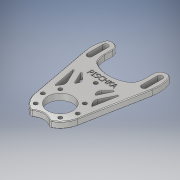
# Autodesk Inventor part: Motor Holder v3
Saved by Autodesk Inventor 2019.4 (Build 234330000, 330)
## iProperties
Created: 2019-03-01
Part Number: Motor Holder v3
Material: Aluminum 6061-AHC
Document SubType Name: Modeling
Designer: Petar
Density: 2.7 g/cm^3
Appearance: Aluminum - Dark
Mass: 26.5004 g
Surface Area: 70.5339 cm^2
Volume: 9.81495 cm^3
Author: Petar
Autodesk Inventor part; units mm, degrees
ref_plane "YZ Plane" through (0, 0, 0) normal (1, 0, 0) x (0, 1, 0)
ref_plane "XZ Plane" through (0, 0, 0) normal (0, 1, 0) x (-1, 0, 0)
ref_plane "XY Plane" through (0, 0, 0) normal (0, 0, 1) x (1, 0, 0)
sketch "Sketch1" plane through (0, 0, 0) normal (0, 1, 0) x (-1, 0, 0)
  line L0 (0, 0) -> (0, 51) construction
  circle A0 centre (0, 51) radius 10
  line L1 (16, -6.25) -> (16, 0)
  line L2 (21.5, 19.954117) -> (21.5, -14.045883) construction
  line L3 (-21.5, 18) -> (-21.5, -16) construction
  circle A1 centre (21.5, 3.5) radius 1.75 construction
  circle A2 centre (21.5, -3.5) radius 1.75 construction
  circle A3 centre (-21.5, 3.5) radius 1.75 construction
  circle A4 centre (-21.5, -3.5) radius 1.75 construction
  line L4 (-16, -6.25) -> (-16, 0)
  line L5 (21.5, 6.25) -> (21.5, -6.25) construction
  line L6 (19.45, 6.25) -> (19.45, -6.25)
  line L7 (23.55, -6.25) -> (23.55, 6.25)
  arc A5 (23.55, 6.25) -> (19.45, 6.25) centre (21.5, 6.25) ccw
  arc A6 (19.45, -6.25) -> (23.55, -6.25) centre (21.5, -6.25) ccw
  line L8 (-19.45, 6.25) -> (-19.45, -6.25)
  line L9 (-23.55, -6.25) -> (-23.55, 6.25)
  arc A7 (-19.45, 6.25) -> (-23.55, 6.25) centre (-21.5, 6.25) ccw
  arc A8 (-23.55, -6.25) -> (-19.45, -6.25) centre (-21.5, -6.25) ccw
  arc A9 (14.562609, 41.295341) -> (17.19371, 54.259804) centre (0, 51) ccw construction
  arc A10 (16, -6.25) -> (24.816002, -10.637953) centre (21.5, -6.25) ccw
  arc A11 (-24.816002, -10.637953) -> (-16, -6.25) centre (-21.5, -6.25) ccw
  line L10 (17.19371, 54.259804) -> (26.527439, 5.029412)
  line L11 (-17.19371, 54.259804) -> (-26.527439, 5.029412)
  circle A12 centre (0, 51) radius 13.75 construction
  circle A13 centre (9.722718, 60.722718) radius 1.5
  circle A14 centre (9.722718, 41.277282) radius 1.5
  line L12 (0, 51) -> (9.722718, 60.722718) construction
  line L13 (9.722718, 41.277282) -> (0, 51) construction
  circle A15 centre (-9.722718, 60.722718) radius 1.5
  circle A16 centre (-9.722718, 41.277282) radius 1.5
  circle A17 centre (13.75, 51) radius 1.5
  line L14 (13.75, 51) -> (0, 51) construction
  circle A18 centre (-13.75, 51) radius 1.5
  circle A19 centre (0, 22.976561) radius 1.5
  line L15 (14.562609, 41.295341) -> (18.699293, 19.476561)
  arc A20 (17.19371, 54.259804) -> (-17.19371, 54.259804) centre (0, 51) ccw
  arc A21 (-17.19371, 54.259804) -> (-14.562609, 41.295341) centre (0, 51) ccw construction
  line L16 (-14.562609, 41.295341) -> (-18.699293, 19.476561)
  line L17 (7.5, 66.811388) -> (0, 61) construction
  line L18 (0, 61) -> (-7.5, 66.811388) construction
  spline S0 degree 2 poles (7.5, 66.811388) (0, 61) (-7.5, 66.811388) knots 1 1 1 2 2 2
  line L19 (7.5, 66.811388) -> (-7.5, 66.811388) construction
  line L20 (18.699293, 19.476561) -> (-18.699293, 19.476561) construction
  line L21 (18.699293, 19.476561) -> (11.899653, 33.58283)
  line L22 (14.562609, 41.295341) -> (12.187745, 37.73167)
  arc A22 (12.187745, 37.73167) -> (11.899653, 33.58283) centre (15.679416, 35.404788) ccw
  line L23 (-18.699293, 19.476561) -> (-11.899653, 33.58283)
  line L24 (-14.562609, 41.295341) -> (-12.187745, 37.73167)
  arc A23 (-11.899653, 33.58283) -> (-12.187745, 37.73167) centre (-15.679416, 35.404788) ccw
  line L25 (14.258838, 19.476561) -> (8.283423, 31.872924)
  line L26 (14.258838, 19.476561) -> (7.634459, 25.898167)
  line L27 (8.283423, 31.872924) -> (7.173527, 30.207438)
  arc A24 (7.173527, 30.207438) -> (7.634459, 25.898167) centre (9.991429, 28.329562) ccw
  line L28 (-14.258838, 19.476561) -> (-8.283423, 31.872924)
  line L29 (-14.258838, 19.476561) -> (-7.634459, 25.898167)
  line L30 (-8.283423, 31.872924) -> (-7.173527, 30.207438)
  arc A25 (-7.634459, 25.898167) -> (-7.173527, 30.207438) centre (-9.991429, 28.329562) ccw
  arc A26 (24.816002, -10.637953) -> (27, 0) centre (0, 0) ccw
  arc A27 (-24.816002, -10.637953) -> (24.816002, -10.637953) centre (0, 0) ccw construction
  arc A28 (-10.301604, 24.957503) -> (-26.527439, 5.029412) centre (0, 0) ccw construction
  line L31 (21.5, -11.75) -> (-21.5, -11.75) construction
  line L32 (-21.213203, 68.5) -> (25, 68.5) construction
  line L33 (0, 61) -> (0, 61) construction
  arc A29 (13.760985, 8.163043) -> (-13.760985, 8.163043) centre (0, -11.5) ccw
  line L34 (13.760985, 8.163043) -> (-13.760985, 8.163043) construction
  arc A30 (16, 0) -> (13.760985, 8.163043) centre (0, 0) ccw
  arc A31 (-13.760985, 8.163043) -> (-16, 0) centre (0, 0) ccw
  arc A32 (27, 0) -> (26.527439, 5.029412) centre (0, 0) ccw
  arc A33 (-27, 0) -> (-24.816002, -10.637953) centre (0, 0) ccw
  arc A34 (-26.527439, 5.029412) -> (-27, 0) centre (0, 0) ccw
  arc A35 (26.527439, 5.029412) -> (-11.984726, 24.194345) centre (0, 0) ccw construction
  line L35 (16, 0) -> (-16, 0) construction
  point P0 (21.5, 0)
  point P1 (0, 12.5)
  dimension "d1" = 20
  dimension "d0" = 51
  dimension "d3" = 3.5
  dimension "d4" = 3.5
  dimension "d5" = 7
  dimension "d9" = 3.5
  dimension "d11" = 32
  dimension "d15" = 4.1
  dimension "d24" = 3
  dimension "d25" = 3
  dimension "d27" = 45
  dimension "d29" = 3
  dimension "d30" = 3
  dimension "d50" = 15
  dimension "d53" = 27
  dimension "d75" = 80.25
  dimension "d76" = 7.5
  dimension "d77" = 3.75
  dimension "d78" = 0
  dimension "d81" = 6.25
  dimension "d82" = 12.5
  dimension "d85" = 5
  dimension "d86" = 4
  dimension "d98" = 15
  dimension "d99" = 24
  dimension "d101" = 43
  dimension "d104" = 2
  constraints: 70 end point, 58 point on circle, 35 centre point, 26 symmetric about line, 19 tangent, 13 point on line, 7 coincident, 5 horizontal, 5 vertical, 3 parallel, 2 perpendicular, 1 collinear, 1 midpoint, 1 vertical alignment, 16 other
  measures "d0" distance of L0.start L0.end
  measures "d3" diameter of A1
  measures "d4" diameter of A2
  measures "d5" distance of A2.centre A1.centre
  measures "d9" vertical distance of L0.start A1.centre
  measures "d11" distance between parallel lines of L4 L1
  measures "d15" distance between parallel lines of L6 L7
  measures "d24" diameter of A13
  measures "d25" diameter of A14
  measures "d27" angle of L0 L13
  measures "d29" diameter of A17
  measures "d30" diameter of A19
  measures "d50" distance of L17.start L18.end
  measures "d53" radius of A26
  measures "d75" distance between parallel lines of L31 L32
  measures "d78" distance of L33.start L33.end
  measures "d81" vertical distance of L5.start point (0, 12.5)
  measures "d82" distance of L5.end L5.start
  measures "d85" distance between parallel lines of L10 L15
  measures "d86" distance between parallel lines of L21 L25
  measures "d98" angle of L15 L21
  measures "d99" radius of A29
  measures "d101" distance of A4.centre A2.centre
  measures "d104" distance edge to line of A19 L20
extrude "Extrusion3" add sketch "Sketch1" along normal blind 5 contours L1 A30 A29 A31 L4 A11 A33 A34 L11 A20 S0 L10 A32 A26 A10
thread "Thread1" size "M3x0.5" class "6H" standard "ANSI Metric M Profile" full length
thread "Thread2" size "M3x0.5" class "6H" standard "ANSI Metric M Profile" full length
thread "Thread3" size "M3x0.5" class "6H" standard "ANSI Metric M Profile" full length
thread "Thread4" size "M3x0.5" class "6H" standard "ANSI Metric M Profile" full length
thread "Thread5" size "M3x0.5" class "6H" standard "ANSI Metric M Profile" full length
thread "Thread6" size "M3x0.5" class "6H" standard "ANSI Metric M Profile" full length
thread "Thread7" size "M3x0.5" class "6H" standard "ANSI Metric M Profile" full length
sketch "Sketch3" plane through (0, 5, 0) normal (0, 1, 0) x (1, 0, 0)
  line L0 (-12.5, -14.976561) -> (12.5, -14.976561) construction
  line L1 (12.5, -14.976561) -> (12.5, -19.976561) construction
  line L2 (12.5, -19.976561) -> (-12.5, -19.976561) construction
  line L3 (-12.5, -19.976561) -> (-12.5, -14.976561) construction
  line L4 (0, 0) -> (0, -51) construction
  circle A0 centre (0, -22.976561) radius 1.5
  circle A1 centre (0, -51) radius 10 construction
  arc A2 (-24.816002, 10.637953) -> (-26.527439, -5.029412) centre (0, 0) ccw construction
  spline S0 degree 2 poles (-7.943274, -16.682396) (-7.943274, -16.941715) (-8.128039, -17.40849) (-8.293355, -17.570565) knots 0 0 0 1 2 2 2
  spline S1 degree 2 poles (-8.293355, -17.570565) (-8.500811, -17.774779) (-9.061589, -17.985475) (-9.489465, -17.985475) knots 0 0 0 1 2 2 2
  line L5 (-9.489465, -17.985475) -> (-9.940033, -17.985475)
  line L6 (-9.940033, -17.985475) -> (-9.940033, -19.476561)
  line L7 (-9.940033, -19.476561) -> (-10.471637, -19.476561)
  line L8 (-10.471637, -19.476561) -> (-10.471637, -15.476561)
  line L9 (-10.471637, -15.476561) -> (-9.466775, -15.476561)
  spline S2 degree 2 poles (-9.466775, -15.476561) (-9.110211, -15.476561) (-8.611021, -15.593255) (-8.419773, -15.726156) knots 0 0 0 1 2 2 2
  spline S3 degree 2 poles (-8.419773, -15.726156) (-8.19611, -15.878506) (-7.943274, -16.348522) (-7.943274, -16.682396) knots 0 0 0 1 2 2 2
  spline S4 degree 2 poles (-8.497569, -16.698603) (-8.497569, -16.491148) (-8.640195, -16.186448) (-8.786062, -16.089203) knots 0 0 0 1 2 2 2
  spline S5 degree 2 poles (-8.786062, -16.089203) (-8.91248, -16.004924) (-9.249595, -15.936853) (-9.49919, -15.936853) knots 0 0 0 1 2 2 2
  line L10 (-9.49919, -15.936853) -> (-9.940033, -15.936853)
  line L11 (-9.940033, -15.936853) -> (-9.940033, -17.531667)
  line L12 (-9.940033, -17.531667) -> (-9.576986, -17.531667)
  spline S6 degree 2 poles (-9.576986, -17.531667) (-9.252837, -17.531667) (-8.854133, -17.427939) (-8.724474, -17.291796) knots 0 0 0 1 2 2 2
  spline S7 degree 2 poles (-8.724474, -17.291796) (-8.604538, -17.171861) (-8.497569, -16.889851) (-8.497569, -16.698603) knots 0 0 0 1 2 2 2
  line L13 (-6.04376, -19.476561) -> (-7.593193, -19.476561)
  line L14 (-7.593193, -19.476561) -> (-7.593193, -19.068133)
  line L15 (-7.593193, -19.068133) -> (-7.084279, -19.068133)
  line L16 (-7.084279, -19.068133) -> (-7.084279, -15.884989)
  line L17 (-7.084279, -15.884989) -> (-7.593193, -15.884989)
  line L18 (-7.593193, -15.884989) -> (-7.593193, -15.476561)
  line L19 (-7.593193, -15.476561) -> (-6.04376, -15.476561)
  line L20 (-6.04376, -15.476561) -> (-6.04376, -15.884989)
  line L21 (-6.04376, -15.884989) -> (-6.552674, -15.884989)
  line L22 (-6.552674, -15.884989) -> (-6.552674, -19.068133)
  line L23 (-6.552674, -19.068133) -> (-6.04376, -19.068133)
  line L24 (-6.04376, -19.068133) -> (-6.04376, -19.476561)
  spline S8 degree 2 poles (-4.270665, -19.547874) (-4.705025, -19.547874) (-5.314425, -19.366351) (-5.583469, -19.236691) knots 0 0 0 1 2 2 2
  line L25 (-5.583469, -19.236691) -> (-5.583469, -18.568944)
  line L26 (-5.583469, -18.568944) -> (-5.544571, -18.568944)
  spline S9 degree 2 poles (-5.544571, -18.568944) (-5.28201, -18.815297) (-4.617504, -19.087582) (-4.309563, -19.087582) knots 0 0 0 1 2 2 2
  spline S10 degree 2 poles (-4.309563, -19.087582) (-3.86872, -19.087582) (-3.418153, -18.721294) (-3.418153, -18.419835) knots 0 0 0 1 2 2 2
  spline S11 degree 2 poles (-3.418153, -18.419835) (-3.418153, -18.179965) (-3.654781, -17.881748) (-3.910859, -17.807193) knots 0 0 0 1 2 2 2
  spline S12 degree 2 poles (-3.910859, -17.807193) (-4.095624, -17.75533) (-4.403566, -17.684017) (-4.633712, -17.62567) knots 0 0 0 1 2 2 2
  spline S13 degree 2 poles (-4.633712, -17.62567) (-4.841167, -17.570565) (-5.168558, -17.405249) (-5.294976, -17.272347) knots 0 0 0 1 2 2 2
  spline S14 degree 2 poles (-5.294976, -17.272347) (-5.418153, -17.139446) (-5.554295, -16.782882) (-5.554295, -16.549495) knots 0 0 0 1 2 2 2
  spline S15 degree 2 poles (-5.554295, -16.549495) (-5.554295, -16.063271) (-4.795786, -15.405248) (-4.209076, -15.405248) knots 0 0 0 1 2 2 2
  spline S16 degree 2 poles (-4.209076, -15.405248) (-3.871961, -15.405248) (-3.275527, -15.53815) (-3.019449, -15.664568) knots 0 0 0 1 2 2 2
  line L27 (-3.019449, -15.664568) -> (-3.019449, -16.2999)
  line L28 (-3.019449, -16.2999) -> (-3.058347, -16.2999)
  spline S17 degree 2 poles (-3.058347, -16.2999) (-3.249595, -16.12486) (-3.846029, -15.86554) (-4.17342, -15.86554) knots 0 0 0 1 2 2 2
  spline S18 degree 2 poles (-4.17342, -15.86554) (-4.54295, -15.86554) (-5, -16.21238) (-5, -16.49439) knots 0 0 0 1 2 2 2
  spline S19 degree 2 poles (-5, -16.49439) (-5, -16.747226) (-4.730956, -17.048684) (-4.47812, -17.116756) knots 0 0 0 1 2 2 2
  spline S20 degree 2 poles (-4.47812, -17.116756) (-4.309563, -17.162137) (-3.820097, -17.27883) (-3.658023, -17.327453) knots 0 0 0 1 2 2 2
  spline S21 degree 2 poles (-3.658023, -17.327453) (-3.246354, -17.453871) (-2.863858, -17.962785) (-2.863858, -18.335556) knots 0 0 0 1 2 2 2
  spline S22 degree 2 poles (-2.863858, -18.335556) (-2.863858, -18.572185) (-3.055106, -19.025994) (-3.226905, -19.184827) knots 0 0 0 1 2 2 2
  spline S23 degree 2 poles (-3.226905, -19.184827) (-3.418153, -19.359868) (-3.904376, -19.547874) (-4.270665, -19.547874) knots 0 0 0 1 2 2 2
  spline S24 degree 2 poles (-0.76013, -19.547874) (-1.149109, -19.547874) (-1.807131, -19.285313) (-2.047002, -19.022753) knots 0 0 0 1 2 2 2
  spline S25 degree 2 poles (-2.047002, -19.022753) (-2.286872, -18.763433) (-2.549433, -17.985475) (-2.549433, -17.479803) knots 0 0 0 1 2 2 2
  spline S26 degree 2 poles (-2.549433, -17.479803) (-2.549433, -16.977372) (-2.293355, -16.231829) (-2.050243, -15.956302) knots 0 0 0 1 2 2 2
  spline S27 degree 2 poles (-2.050243, -15.956302) (-1.810373, -15.687258) (-1.155592, -15.405248) (-0.750405, -15.405248) knots 0 0 0 1 2 2 2
  spline S28 degree 2 poles (-0.750405, -15.405248) (-0.549433, -15.405248) (-0.19611, -15.463595) (-0.047002, -15.508976) knots 0 0 0 1 2 2 2
  spline S29 degree 2 poles (-0.047002, -15.508976) (0.082658, -15.551116) (0.351702, -15.671051) (0.484603, -15.742364) knots 0 0 0 1 2 2 2
  line L29 (0.484603, -15.742364) -> (0.484603, -16.384179)
  line L30 (0.484603, -16.384179) -> (0.442463, -16.384179)
  spline S30 degree 2 poles (0.442463, -16.384179) (0.371151, -16.319349) (0.150729, -16.137825) (-0.008104, -16.050305) knots 0 0 0 1 2 2 2
  spline S31 degree 2 poles (-0.008104, -16.050305) (-0.160454, -15.966026) (-0.520259, -15.859057) (-0.753647, -15.859057) knots 0 0 0 1 2 2 2
  spline S32 degree 2 poles (-0.753647, -15.859057) (-1.009725, -15.859057) (-1.466775, -16.069754) (-1.638574, -16.270727) knots 0 0 0 1 2 2 2
  spline S33 degree 2 poles (-1.638574, -16.270727) (-1.807131, -16.474941) (-1.995138, -17.094065) (-1.995138, -17.479803) knots 0 0 0 1 2 2 2
  spline S34 degree 2 poles (-1.995138, -17.479803) (-1.995138, -17.891472) (-1.797407, -18.484665) (-1.625608, -18.688879) knots 0 0 0 1 2 2 2
  spline S35 degree 2 poles (-1.625608, -18.688879) (-1.45705, -18.88661) (-1.006483, -19.087582) (-0.753647, -19.087582) knots 0 0 0 1 2 2 2
  spline S36 degree 2 poles (-0.753647, -19.087582) (-0.523501, -19.087582) (-0.131281, -18.97413) (0.02107, -18.889851) knots 0 0 0 1 2 2 2
  spline S37 degree 2 poles (0.02107, -18.889851) (0.166937, -18.805573) (0.384117, -18.630532) (0.445705, -18.568944) knots 0 0 0 1 2 2 2
  line L31 (0.445705, -18.568944) -> (0.484603, -18.568944)
  line L32 (0.484603, -18.568944) -> (0.484603, -19.204276)
  spline S38 degree 2 poles (0.484603, -19.204276) (0.351702, -19.265864) (0.118314, -19.379317) (-0.047002, -19.43118) knots 0 0 0 1 2 2 2
  spline S39 degree 2 poles (-0.047002, -19.43118) (-0.222042, -19.489527) (-0.520259, -19.547874) (-0.76013, -19.547874) knots 0 0 0 1 2 2 2
  line L33 (3.884927, -19.476561) -> (3.353322, -19.476561)
  line L34 (3.353322, -19.476561) -> (3.353322, -17.518701)
  line L35 (3.353322, -17.518701) -> (1.512155, -17.518701)
  line L36 (1.512155, -17.518701) -> (1.512155, -19.476561)
  line L37 (1.512155, -19.476561) -> (0.980551, -19.476561)
  line L38 (0.980551, -19.476561) -> (0.980551, -15.476561)
  line L39 (0.980551, -15.476561) -> (1.512155, -15.476561)
  line L40 (1.512155, -15.476561) -> (1.512155, -17.045443)
  line L41 (1.512155, -17.045443) -> (3.353322, -17.045443)
  line L42 (3.353322, -17.045443) -> (3.353322, -15.476561)
  line L43 (3.353322, -15.476561) -> (3.884927, -15.476561)
  line L44 (3.884927, -15.476561) -> (3.884927, -19.476561)
  line L45 (7.612642, -19.476561) -> (6.922204, -19.476561)
  line L46 (6.922204, -19.476561) -> (5.460292, -17.615945)
  line L47 (5.460292, -17.615945) -> (5.226904, -17.878506)
  line L48 (5.226904, -17.878506) -> (5.226904, -19.476561)
  line L49 (5.226904, -19.476561) -> (4.6953, -19.476561)
  line L50 (4.6953, -19.476561) -> (4.6953, -15.476561)
  line L51 (4.6953, -15.476561) -> (5.226904, -15.476561)
  line L52 (5.226904, -15.476561) -> (5.226904, -17.314487)
  line L53 (5.226904, -17.314487) -> (6.867099, -15.476561)
  line L54 (6.867099, -15.476561) -> (7.515397, -15.476561)
  line L55 (7.515397, -15.476561) -> (5.858995, -17.262623)
  line L56 (5.858995, -17.262623) -> (7.612642, -19.476561)
  line L57 (7.49919, -19.476561) -> (8.84765, -15.476561)
  line L58 (8.84765, -15.476561) -> (9.502431, -15.476561)
  line L59 (9.502431, -15.476561) -> (10.850891, -19.476561)
  line L60 (10.850891, -19.476561) -> (10.290113, -19.476561)
  line L61 (10.290113, -19.476561) -> (9.927066, -18.358247)
  line L62 (9.927066, -18.358247) -> (8.400324, -18.358247)
  line L63 (8.400324, -18.358247) -> (8.037277, -19.476561)
  line L64 (8.037277, -19.476561) -> (7.49919, -19.476561)
  line L65 (9.781199, -17.904438) -> (9.162075, -16.021132)
  line L66 (9.162075, -16.021132) -> (8.546191, -17.904438)
  line L67 (8.546191, -17.904438) -> (9.781199, -17.904438)
  dimension "d68" = 3
  dimension "d69" = 5
  dimension "d70" = 25
  constraints: 2 coincident, 2 end point, 1 vertical, 3 other
  measures "d68" distance from line of L2 A0.centre
  measures "d69" distance between parallel lines of L0 L2
  measures "d70" distance between parallel lines of L3 L1
emboss "Emboss1" sketch "Sketch3" operation cut depth 0.2 direction (0, -1, 0) contours S0 S1 L5 L6 L7 L8 L9 S2 S3 | L13 L14 L15 L16 L17 L18 L19 L20 L21 L22 L23 L24 | S8 L25 L26 S9 S10 S11 S12 S13 S14 S15 S16 L27 L28 S17 S18 S19 S20 S21 S22 S23 | S24 S25 S26 S27 S28 S29 L29 L30 S30 S31 S32 S33 S34 S35 S36 S37 L31 L32 S38 S39 | L33 L34 L35 L36 L37 L38 L39 L40 L41 L42 L43 L44 | L45 L57 L56 | L56 L57 L58 L59 L60 L61 L62 L63 L64 | L45 L46 L47 L48 L49 L50 L51 L52 L53 L54 L55 L56 L57
sketch "Sketch4" plane through (0, 0, 0) normal (0, -1, 0) x (1, 0, 0)
  circle A0 centre (0, 22.976561) radius 1.5
  line L0 (12.5, 14.976561) -> (-12.5, 14.976561) construction
  line L1 (-12.5, 14.976561) -> (-12.5, 19.976561) construction
  line L2 (-12.5, 19.976561) -> (12.5, 19.976561) construction
  line L3 (12.5, 19.976561) -> (12.5, 14.976561) construction
  circle A1 centre (0, 51) radius 10 construction
  arc A2 (24.816002, -10.637953) -> (26.527439, 5.029412) centre (0, 0) ccw construction
  line L4 (0, 0) -> (0, 51) construction
  spline S0 degree 2 poles (7.943274, 16.682396) (7.943274, 16.941715) (8.128039, 17.40849) (8.293355, 17.570565) knots 0 0 0 1 2 2 2
  spline S1 degree 2 poles (8.293355, 17.570565) (8.500811, 17.774779) (9.061589, 17.985475) (9.489465, 17.985475) knots 0 0 0 1 2 2 2
  line L5 (9.489465, 17.985475) -> (9.940033, 17.985475)
  line L6 (9.940033, 17.985475) -> (9.940033, 19.476561)
  line L7 (9.940033, 19.476561) -> (10.471637, 19.476561)
  line L8 (10.471637, 19.476561) -> (10.471637, 15.476561)
  line L9 (10.471637, 15.476561) -> (9.466775, 15.476561)
  spline S2 degree 2 poles (9.466775, 15.476561) (9.110211, 15.476561) (8.611021, 15.593255) (8.419773, 15.726156) knots 0 0 0 1 2 2 2
  spline S3 degree 2 poles (8.419773, 15.726156) (8.19611, 15.878506) (7.943274, 16.348522) (7.943274, 16.682396) knots 0 0 0 1 2 2 2
  spline S4 degree 2 poles (8.497569, 16.698603) (8.497569, 16.491148) (8.640195, 16.186448) (8.786062, 16.089203) knots 0 0 0 1 2 2 2
  spline S5 degree 2 poles (8.786062, 16.089203) (8.91248, 16.004924) (9.249595, 15.936853) (9.49919, 15.936853) knots 0 0 0 1 2 2 2
  line L10 (9.49919, 15.936853) -> (9.940033, 15.936853)
  line L11 (9.940033, 15.936853) -> (9.940033, 17.531667)
  line L12 (9.940033, 17.531667) -> (9.576986, 17.531667)
  spline S6 degree 2 poles (9.576986, 17.531667) (9.252837, 17.531667) (8.854133, 17.427939) (8.724474, 17.291796) knots 0 0 0 1 2 2 2
  spline S7 degree 2 poles (8.724474, 17.291796) (8.604538, 17.171861) (8.497569, 16.889851) (8.497569, 16.698603) knots 0 0 0 1 2 2 2
  line L13 (6.04376, 19.476561) -> (7.593193, 19.476561)
  line L14 (7.593193, 19.476561) -> (7.593193, 19.068133)
  line L15 (7.593193, 19.068133) -> (7.084279, 19.068133)
  line L16 (7.084279, 19.068133) -> (7.084279, 15.884989)
  line L17 (7.084279, 15.884989) -> (7.593193, 15.884989)
  line L18 (7.593193, 15.884989) -> (7.593193, 15.476561)
  line L19 (7.593193, 15.476561) -> (6.04376, 15.476561)
  line L20 (6.04376, 15.476561) -> (6.04376, 15.884989)
  line L21 (6.04376, 15.884989) -> (6.552674, 15.884989)
  line L22 (6.552674, 15.884989) -> (6.552674, 19.068133)
  line L23 (6.552674, 19.068133) -> (6.04376, 19.068133)
  line L24 (6.04376, 19.068133) -> (6.04376, 19.476561)
  spline S8 degree 2 poles (4.270665, 19.547874) (4.705025, 19.547874) (5.314425, 19.366351) (5.583469, 19.236691) knots 0 0 0 1 2 2 2
  line L25 (5.583469, 19.236691) -> (5.583469, 18.568944)
  line L26 (5.583469, 18.568944) -> (5.544571, 18.568944)
  spline S9 degree 2 poles (5.544571, 18.568944) (5.28201, 18.815297) (4.617504, 19.087582) (4.309563, 19.087582) knots 0 0 0 1 2 2 2
  spline S10 degree 2 poles (4.309563, 19.087582) (3.86872, 19.087582) (3.418153, 18.721294) (3.418153, 18.419835) knots 0 0 0 1 2 2 2
  spline S11 degree 2 poles (3.418153, 18.419835) (3.418153, 18.179965) (3.654781, 17.881748) (3.910859, 17.807193) knots 0 0 0 1 2 2 2
  spline S12 degree 2 poles (3.910859, 17.807193) (4.095624, 17.75533) (4.403566, 17.684017) (4.633712, 17.62567) knots 0 0 0 1 2 2 2
  spline S13 degree 2 poles (4.633712, 17.62567) (4.841167, 17.570565) (5.168558, 17.405249) (5.294976, 17.272347) knots 0 0 0 1 2 2 2
  spline S14 degree 2 poles (5.294976, 17.272347) (5.418153, 17.139446) (5.554295, 16.782882) (5.554295, 16.549495) knots 0 0 0 1 2 2 2
  spline S15 degree 2 poles (5.554295, 16.549495) (5.554295, 16.063271) (4.795786, 15.405248) (4.209076, 15.405248) knots 0 0 0 1 2 2 2
  spline S16 degree 2 poles (4.209076, 15.405248) (3.871961, 15.405248) (3.275527, 15.53815) (3.019449, 15.664568) knots 0 0 0 1 2 2 2
  line L27 (3.019449, 15.664568) -> (3.019449, 16.2999)
  line L28 (3.019449, 16.2999) -> (3.058347, 16.2999)
  spline S17 degree 2 poles (3.058347, 16.2999) (3.249595, 16.12486) (3.846029, 15.86554) (4.17342, 15.86554) knots 0 0 0 1 2 2 2
  spline S18 degree 2 poles (4.17342, 15.86554) (4.54295, 15.86554) (5, 16.21238) (5, 16.49439) knots 0 0 0 1 2 2 2
  spline S19 degree 2 poles (5, 16.49439) (5, 16.747226) (4.730956, 17.048684) (4.47812, 17.116756) knots 0 0 0 1 2 2 2
  spline S20 degree 2 poles (4.47812, 17.116756) (4.309563, 17.162137) (3.820097, 17.27883) (3.658023, 17.327453) knots 0 0 0 1 2 2 2
  spline S21 degree 2 poles (3.658023, 17.327453) (3.246354, 17.453871) (2.863858, 17.962785) (2.863858, 18.335556) knots 0 0 0 1 2 2 2
  spline S22 degree 2 poles (2.863858, 18.335556) (2.863858, 18.572185) (3.055106, 19.025994) (3.226905, 19.184827) knots 0 0 0 1 2 2 2
  spline S23 degree 2 poles (3.226905, 19.184827) (3.418153, 19.359868) (3.904376, 19.547874) (4.270665, 19.547874) knots 0 0 0 1 2 2 2
  spline S24 degree 2 poles (0.76013, 19.547874) (1.149109, 19.547874) (1.807131, 19.285313) (2.047002, 19.022753) knots 0 0 0 1 2 2 2
  spline S25 degree 2 poles (2.047002, 19.022753) (2.286872, 18.763433) (2.549433, 17.985475) (2.549433, 17.479803) knots 0 0 0 1 2 2 2
  spline S26 degree 2 poles (2.549433, 17.479803) (2.549433, 16.977372) (2.293355, 16.231829) (2.050243, 15.956302) knots 0 0 0 1 2 2 2
  spline S27 degree 2 poles (2.050243, 15.956302) (1.810373, 15.687258) (1.155592, 15.405248) (0.750405, 15.405248) knots 0 0 0 1 2 2 2
  spline S28 degree 2 poles (0.750405, 15.405248) (0.549433, 15.405248) (0.19611, 15.463595) (0.047002, 15.508976) knots 0 0 0 1 2 2 2
  spline S29 degree 2 poles (0.047002, 15.508976) (-0.082658, 15.551116) (-0.351702, 15.671051) (-0.484603, 15.742364) knots 0 0 0 1 2 2 2
  line L29 (-0.484603, 15.742364) -> (-0.484603, 16.384179)
  line L30 (-0.484603, 16.384179) -> (-0.442463, 16.384179)
  spline S30 degree 2 poles (-0.442463, 16.384179) (-0.371151, 16.319349) (-0.150729, 16.137825) (0.008104, 16.050305) knots 0 0 0 1 2 2 2
  spline S31 degree 2 poles (0.008104, 16.050305) (0.160454, 15.966026) (0.520259, 15.859057) (0.753647, 15.859057) knots 0 0 0 1 2 2 2
  spline S32 degree 2 poles (0.753647, 15.859057) (1.009725, 15.859057) (1.466775, 16.069754) (1.638574, 16.270727) knots 0 0 0 1 2 2 2
  spline S33 degree 2 poles (1.638574, 16.270727) (1.807131, 16.474941) (1.995138, 17.094065) (1.995138, 17.479803) knots 0 0 0 1 2 2 2
  spline S34 degree 2 poles (1.995138, 17.479803) (1.995138, 17.891472) (1.797407, 18.484665) (1.625608, 18.688879) knots 0 0 0 1 2 2 2
  spline S35 degree 2 poles (1.625608, 18.688879) (1.45705, 18.88661) (1.006483, 19.087582) (0.753647, 19.087582) knots 0 0 0 1 2 2 2
  spline S36 degree 2 poles (0.753647, 19.087582) (0.523501, 19.087582) (0.131281, 18.97413) (-0.02107, 18.889851) knots 0 0 0 1 2 2 2
  spline S37 degree 2 poles (-0.02107, 18.889851) (-0.166937, 18.805573) (-0.384117, 18.630532) (-0.445705, 18.568944) knots 0 0 0 1 2 2 2
  line L31 (-0.445705, 18.568944) -> (-0.484603, 18.568944)
  line L32 (-0.484603, 18.568944) -> (-0.484603, 19.204276)
  spline S38 degree 2 poles (-0.484603, 19.204276) (-0.351702, 19.265864) (-0.118314, 19.379317) (0.047002, 19.43118) knots 0 0 0 1 2 2 2
  spline S39 degree 2 poles (0.047002, 19.43118) (0.222042, 19.489527) (0.520259, 19.547874) (0.76013, 19.547874) knots 0 0 0 1 2 2 2
  line L33 (-3.884927, 19.476561) -> (-3.353322, 19.476561)
  line L34 (-3.353322, 19.476561) -> (-3.353322, 17.518701)
  line L35 (-3.353322, 17.518701) -> (-1.512155, 17.518701)
  line L36 (-1.512155, 17.518701) -> (-1.512155, 19.476561)
  line L37 (-1.512155, 19.476561) -> (-0.980551, 19.476561)
  line L38 (-0.980551, 19.476561) -> (-0.980551, 15.476561)
  line L39 (-0.980551, 15.476561) -> (-1.512155, 15.476561)
  line L40 (-1.512155, 15.476561) -> (-1.512155, 17.045443)
  line L41 (-1.512155, 17.045443) -> (-3.353322, 17.045443)
  line L42 (-3.353322, 17.045443) -> (-3.353322, 15.476561)
  line L43 (-3.353322, 15.476561) -> (-3.884927, 15.476561)
  line L44 (-3.884927, 15.476561) -> (-3.884927, 19.476561)
  line L45 (-7.612642, 19.476561) -> (-6.922204, 19.476561)
  line L46 (-6.922204, 19.476561) -> (-5.460292, 17.615945)
  line L47 (-5.460292, 17.615945) -> (-5.226904, 17.878506)
  line L48 (-5.226904, 17.878506) -> (-5.226904, 19.476561)
  line L49 (-5.226904, 19.476561) -> (-4.6953, 19.476561)
  line L50 (-4.6953, 19.476561) -> (-4.6953, 15.476561)
  line L51 (-4.6953, 15.476561) -> (-5.226904, 15.476561)
  line L52 (-5.226904, 15.476561) -> (-5.226904, 17.314487)
  line L53 (-5.226904, 17.314487) -> (-6.867099, 15.476561)
  line L54 (-6.867099, 15.476561) -> (-7.515397, 15.476561)
  line L55 (-7.515397, 15.476561) -> (-5.858995, 17.262623)
  line L56 (-5.858995, 17.262623) -> (-7.612642, 19.476561)
  line L57 (-7.49919, 19.476561) -> (-8.84765, 15.476561)
  line L58 (-8.84765, 15.476561) -> (-9.502431, 15.476561)
  line L59 (-9.502431, 15.476561) -> (-10.850891, 19.476561)
  line L60 (-10.850891, 19.476561) -> (-10.290113, 19.476561)
  line L61 (-10.290113, 19.476561) -> (-9.927066, 18.358247)
  line L62 (-9.927066, 18.358247) -> (-8.400324, 18.358247)
  line L63 (-8.400324, 18.358247) -> (-8.037277, 19.476561)
  line L64 (-8.037277, 19.476561) -> (-7.49919, 19.476561)
  line L65 (-9.781199, 17.904438) -> (-9.162075, 16.021132)
  line L66 (-9.162075, 16.021132) -> (-8.546191, 17.904438)
  line L67 (-8.546191, 17.904438) -> (-9.781199, 17.904438)
  dimension "d67" = 3
  dimension "d71" = 5
  dimension "d72" = 25
  constraints: 2 end point, 1 vertical, 3 other
  measures "d67" distance from line of L2 A0.centre
  measures "d71" distance between parallel lines of L2 L0
  measures "d72" distance between parallel lines of L3 L1
emboss "Emboss2" sketch "Sketch4" operation cut depth 0.2 direction (0, 1, 0) contours S0 S1 L5 L6 L7 L8 L9 S2 S3 | L13 L14 L15 L16 L17 L18 L19 L20 L21 L22 L23 L24 | S8 L25 L26 S9 S10 S11 S12 S13 S14 S15 S16 L27 L28 S17 S18 S19 S20 S21 S22 S23 | S24 S25 S26 S27 S28 S29 L29 L30 S30 S31 S32 S33 S34 S35 S36 S37 L31 L32 S38 S39 | L33 L34 L35 L36 L37 L38 L39 L40 L41 L42 L43 L44 | L45 L57 L56 | L56 L57 L58 L59 L60 L61 L62 L63 L64 | L45 L46 L47 L48 L49 L50 L51 L52 L53 L54 L55 L56 L57
fillet "Fillet3" radius 0.5 8 edges at (-18.6993, 2.5, 19.4766) (-14.2588, 2.5, 19.4766) (-8.2834, 2.5, 31.8729) (-14.5626, 2.5, 41.2953) (8.2834, 2.5, 31.8729) (14.5626, 2.5, 41.2953) (18.6993, 2.5, 19.4766) (14.2588, 2.5, 19.4766)
fillet "Fillet5" radius 2 6 edges at (-7.5, 2.5, 66.8114) (7.5, 2.5, 66.8114) (24.816, 2.5, -10.638) (-24.816, 2.5, -10.638) (-13.761, 2.5, 8.163) (13.761, 2.5, 8.163)
chamfer "Chamfer3" distance 0.5 angle 45 40 edges at (14.2416, 5, 61.1699) (21.8606, 5, 29.6446) (26.8729, 5, -2.6167) (24.7034, 5, -10.6299) (18.713, 5, -10.9916) (16, 5, -3.125) (15.4929, 5, 3.9962) (13.7269, 5, 8.124) (0, 5, 12.5) (7.5963, 5, 66.4658) (0, 5, 63.9057) (-7.5963, 5, 66.4658) (-14.2416, 5, 61.1699) (-21.8606, 5, 29.6446) (-26.8729, 5, -2.6167) (-24.7034, 5, -10.6299) (-18.713, 5, -10.9916) (-16, 5, -3.125) (-15.4929, 5, 3.9962) (-13.7269, 5, 8.124) (0, 0, 63.9057) (7.5963, 0, 66.4658) (14.2416, 0, 61.1699) (21.8606, 0, 29.6446) (26.8729, 0, -2.6167) (24.7034, 0, -10.6299) (18.713, 0, -10.9916) (16, 0, -3.125) (15.4929, 0, 3.9962) (13.7269, 0, 8.124) (0, 0, 12.5) (-7.5963, 0, 66.4658) (-14.2416, 0, 61.1699) (-21.8606, 0, 29.6446) (-26.8729, 0, -2.6167) (-24.7034, 0, -10.6299) (-18.713, 0, -10.9916) (-16, 0, -3.125) (-15.4929, 0, 3.9962) (-13.7269, 0, 8.124)
sketch "Center Lines" plane through (0, 5, 0) normal (0, 1, 0) x (1, 0, 0)
  arc A0 (-23.55, -6.25) -> (-19.45, -6.25) centre (-21.5, -6.25) ccw construction
  line L0 (-23.55, -6.25) -> (-23.55, 6.25) construction
  arc A1 (-19.45, 6.25) -> (-23.55, 6.25) centre (-21.5, 6.25) ccw construction
  line L1 (-19.45, 6.25) -> (-19.45, -6.25) construction
  line L2 (-21.5, -6.25) -> (-21.5, 6.25) construction
  line L3 (19.45, -6.25) -> (19.45, 6.25) construction
  arc A2 (19.45, -6.25) -> (23.55, -6.25) centre (21.5, -6.25) ccw construction
  line L4 (23.55, 6.25) -> (23.55, -6.25) construction
  arc A3 (23.55, 6.25) -> (19.45, 6.25) centre (21.5, 6.25) ccw construction
  line L5 (21.5, -6.25) -> (21.5, 6.25) construction
  constraints: 4 end point, 2 vertical
body "Solid3"
